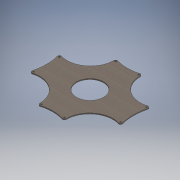
# Autodesk Inventor part: dribler_floor
Saved by Autodesk Inventor 2020 (Build 240168000, 168)
## iProperties
Created: 2024-11-13
Part Number: dribler_floor
Material: Типовые
Document SubType Name: Modeling
Designer: Ivan
Density: 1 g/cm^3
Appearance: Орех
Author: Ivan
Autodesk Inventor part; units mm, degrees
ref_plane "YZ Plane" through (0, 0, 0) normal (1, 0, 0) x (0, 1, 0)
ref_plane "XZ Plane" through (0, 0, 0) normal (0, 1, 0) x (-1, 0, 0)
ref_plane "XY Plane" through (0, 0, 0) normal (0, 0, 1) x (1, 0, 0)
sketch "Эскиз1" plane through (0, 2, -127) normal (0, 1, 0) x (1, 0, 0)
  circle A0 centre (-90.3481, -100.1076) radius 1.5
  circle A1 centre (90.3481, -153.8924) radius 1.5
  circle A2 centre (-90.3481, -153.8924) radius 1.5
  circle A3 centre (90.3481, -100.1076) radius 1.5
  circle A4 centre (51.0265, -155.3991) radius 1.5
  circle A5 centre (-67.0849, -171.4575) radius 1.5
  circle A6 centre (-44.4575, -59.9151) radius 1.5
  circle A7 centre (51.0265, -98.6009) radius 1.5
  circle A8 centre (28.3991, -75.9735) radius 1.5
  circle A9 centre (-67.0849, -82.5425) radius 1.5
  circle A10 centre (-28.3991, -178.0265) radius 1.5
  circle A11 centre (28.3991, -178.0265) radius 1.5
  circle A12 centre (67.0849, -171.4575) radius 1.5
  circle A13 centre (-51.0265, -155.3991) radius 1.5
  circle A14 centre (-28.3991, -75.9735) radius 1.5
  circle A15 centre (67.0849, -82.5425) radius 1.5
  circle A16 centre (44.4575, -59.9151) radius 1.5
  circle A17 centre (-51.0265, -98.6009) radius 1.5
  circle A18 centre (-44.4575, -194.0849) radius 1.5
  circle A19 centre (44.4575, -194.0849) radius 1.5
  arc A20 (-36.9892, -29.8002) -> (36.9892, -29.8002) centre (0, 0) ccw
  arc A21 (-36.9892, -29.8002) -> (-48.2758, -34.8835) centre (0, -127) ccw
  line L0 (-48.2758, -34.8835) -> (-38.4471, -44.7123)
  line L1 (-38.4471, -44.7123) -> (-82.2877, -88.5529)
  line L2 (-82.2877, -88.5529) -> (-92.1165, -78.7242)
  arc A22 (-92.1165, -78.7242) -> (-92.1165, -175.2758) centre (0, -127) ccw
  line L3 (-92.1165, -175.2758) -> (-82.2877, -165.4471)
  line L4 (-82.2877, -165.4471) -> (-38.4471, -209.2877)
  line L5 (-38.4471, -209.2877) -> (-48.2758, -219.1165)
  arc A23 (-48.2758, -219.1165) -> (-36.9892, -224.1998) centre (0, -127) ccw
  arc A24 (36.9892, -224.1998) -> (-36.9892, -224.1998) centre (0, -254) ccw
  arc A25 (36.9892, -224.1998) -> (48.2758, -219.1165) centre (0, -127) ccw
  line L6 (48.2758, -219.1165) -> (38.4471, -209.2877)
  line L7 (38.4471, -209.2877) -> (82.2877, -165.4471)
  line L8 (82.2877, -165.4471) -> (92.1165, -175.2758)
  arc A26 (92.1165, -175.2758) -> (92.1165, -78.7242) centre (0, -127) ccw
  line L9 (92.1165, -78.7242) -> (82.2877, -88.5529)
  line L10 (82.2877, -88.5529) -> (38.4471, -44.7123)
  line L11 (38.4471, -44.7123) -> (48.2758, -34.8835)
  arc A27 (48.2758, -34.8835) -> (36.9892, -29.8002) centre (0, -127) ccw
  line L12 (-67.0849, -82.5425) -> (-51.0265, -98.6009) construction
  circle A28 centre (0, -127) radius 69.3873
  line L13 (-62.0891, -96.0236) -> (-51.0265, -107.0862)
  line L14 (-51.0265, -107.0862) -> (-19.9138, -75.9735)
  line L15 (-19.9138, -75.9735) -> (-30.9764, -64.9109)
  line L16 (-51.0265, -146.9138) -> (-62.0891, -157.9764)
  line L17 (-19.9138, -178.0265) -> (-51.0265, -146.9138)
  line L18 (-30.9764, -189.0891) -> (-19.9138, -178.0265)
  line L19 (19.9138, -178.0265) -> (30.9764, -189.0891)
  line L20 (51.0265, -146.9138) -> (19.9138, -178.0265)
  line L21 (62.0891, -157.9764) -> (51.0265, -146.9138)
  line L22 (51.0265, -107.0862) -> (62.0891, -96.0236)
  line L23 (19.9138, -75.9735) -> (51.0265, -107.0862)
  line L24 (30.9764, -64.9109) -> (19.9138, -75.9735)
  point P0 (-59.0557, -90.5717)
sketch "Эскиз2_1" plane through (0, 2, 127) normal (0, 1, 0) x (1, 0, 0)
  circle A0 centre (0, 127) radius 104
  line L0 (-92.1165, 78.7242) -> (-82.2877, 88.5529)
  line L1 (-82.2877, 88.5529) -> (-38.4471, 44.7123)
  line L2 (-38.4471, 44.7123) -> (-48.2758, 34.8835)
  line L3 (48.2758, 34.8835) -> (38.4471, 44.7123)
  line L4 (38.4471, 44.7123) -> (82.2877, 88.5529)
  line L5 (82.2877, 88.5529) -> (92.1165, 78.7242)
  line L6 (82.2877, 165.4471) -> (38.4471, 209.2877)
  line L7 (38.4471, 209.2877) -> (48.2758, 219.1165)
  line L8 (92.1165, 175.2758) -> (82.2877, 165.4471)
  line L9 (-48.2758, 219.1165) -> (-38.4471, 209.2877)
  line L10 (-38.4471, 209.2877) -> (-82.2877, 165.4471)
  line L11 (-82.2877, 165.4471) -> (-92.1165, 175.2758)
sketch "Эскиз3" plane through (0, 2, 127) normal (0, 1, 0) x (1, 0, 0)
  circle A0 centre (-23.8556, 50.0189) radius 1.5
  circle A1 centre (23.8556, 50.0189) radius 1.5
  circle A2 centre (-23.8556, 203.9811) radius 1.5
  circle A3 centre (23.8556, 203.9811) radius 1.5
  point P0 (0, 127)
sketch "Эскиз6" plane through (0, 0, 0) normal (0, 1, 0) x (-1, 0, 0)
  circle A0 centre (0, 0) radius 49.5
  circle A1 centre (0, 0) radius 41
  dimension "d1" = 99
  dimension "d2" = 82
  constraints: 2 centre point, 2 coincident
  measures "d1" diameter of A0
  measures "d2" diameter of A1
sketch "Эскиз7" plane through (0, 0, 0) normal (0, 1, 0) x (-1, 0, 0)
  circle A0 centre (90.3481, 26.8924) radius 1.5 projected
  circle A1 centre (90.3481, -26.8924) radius 1.5 projected
  circle A2 centre (23.8556, 76.9811) radius 1.5 projected
  circle A3 centre (23.8556, -76.9811) radius 1.5 projected
  circle A4 centre (-23.8556, -76.9811) radius 1.5 projected
  circle A5 centre (-23.8556, 76.9811) radius 1.5 projected
  circle A6 centre (-90.3481, 26.8924) radius 1.5 projected
  circle A7 centre (-90.3481, -26.8924) radius 1.5 projected
  circle A8 centre (0, 0) radius 28
  circle A9 centre (90.3481, 26.8924) radius 3.5
  circle A10 centre (90.3481, -26.8924) radius 3.5
  circle A11 centre (23.8556, -76.9811) radius 3.5
  circle A12 centre (-23.8556, -76.9811) radius 3.5
  circle A13 centre (-90.3481, -26.8924) radius 3.5
  circle A14 centre (-90.3481, 26.8924) radius 3.5
  circle A15 centre (23.8556, 76.9811) radius 3.5
  circle A16 centre (-23.8556, 76.9811) radius 3.5
  line L0 (0, 0) -> (28, 0) construction
  line L1 (23.8556, 76.9811) -> (27.3556, 76.9811) construction
  line L2 (90.3481, 26.8924) -> (90.3481, 30.3924) construction
  arc A17 (27.3556, 76.9811) -> (90.3481, 30.3924) centre (76.0802, 76.9811) ccw
  line L3 (27.3556, 76.9811) -> (27.3556, 30.3924) construction
  line L4 (27.3556, 30.3924) -> (90.3481, 30.3924) construction
  arc A18 (90.3481, -30.3924) -> (27.3556, -76.9811) centre (76.0802, -76.9811) ccw
  line L5 (0, 0) -> (0, 28) construction
  arc A19 (-90.3481, 30.3924) -> (-27.3556, 76.9811) centre (-76.0802, 76.9811) ccw
  arc A20 (-27.3556, -76.9811) -> (-90.3481, -30.3924) centre (-76.0802, -76.9811) ccw
  line L6 (90.3481, 26.8924) -> (93.8481, 26.8924) construction
  line L7 (90.3481, -26.8924) -> (93.8481, -26.8924) construction
  arc A21 (93.8481, 26.8924) -> (93.8481, -26.8924) centre (195.4124, 0) ccw
  arc A22 (-93.8481, -26.8924) -> (-93.8481, 26.8924) centre (-195.4124, 0) ccw
  line L8 (-23.8556, 76.9811) -> (-23.8556, 80.4811) construction
  line L9 (23.8556, 76.9811) -> (23.8556, 80.4811) construction
  arc A23 (-23.8556, 80.4811) -> (23.8556, 80.4811) centre (0, 160.0297) ccw
  arc A24 (23.8556, -80.4811) -> (-23.8556, -80.4811) centre (0, -160.0297) ccw
  point P0 (-27.3556, 76.9811)
  point P1 (-90.3481, 30.3924)
  point P2 (-93.8481, 26.8924)
  point P3 (-93.8481, -26.8924)
  point P4 (-90.3481, -30.3924)
  point P5 (-27.3556, -76.9811)
  point P6 (-23.8556, -80.4811)
  point P7 (23.8556, -80.4811)
  point P8 (90.3481, -30.3924)
  dimension "d3" = 56
  dimension "d4" = 7
  constraints: 22 point on circle, 20 end point, 15 centre point, 15 symmetric about line, 9 coincident, 3 equal radius, 3 horizontal, 3 tangent, 3 vertical, 2 parallel, 2 perpendicular, 15 other
  measures "d3" diameter of A8
  measures "d4" diameter of A9
extrude "Выдавливание1" add sketch "Эскиз7" along normal blind 2 contours A21 A9 A17 | A21 A10 A18 A11 A24 A12 A20 A13 A22 A14 A19 A16 A23 A15 A17 A9 | A21 A10 A18 | A15 A23 | A11 A24 | A16 A23 | A24 A12 | A14 A22 A19 | A20 A13 A22 picked at (26.6398, 76.5793) picked at (26.6398, -76.5793) picked at (-21.0707, 76.5822) picked at (-26.5069, -76.0401)
